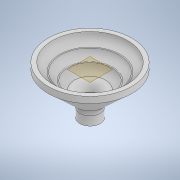
# Autodesk Inventor part: TubeExpander
Saved by Autodesk Inventor 2020 (Build 240168000, 168)
## iProperties
Created: 2020-04-23
Part Number: TubeExpander
Material: Типовые
Document SubType Name: Modeling
Designer: Михаил
Density: 1 g/cm^3
Appearance: По умолчанию
Author: Михаил
Autodesk Inventor part; units mm, degrees
ref_plane "YZ Plane" through (0, 0, 0) normal (1, 0, 0) x (0, 1, 0)
ref_plane "XZ Plane" through (0, 0, 0) normal (0, 1, 0) x (-1, 0, 0)
ref_plane "XY Plane" through (0, 0, 0) normal (0, 0, 1) x (1, 0, 0)
sketch "Эскиз1" plane through (0, 0, 0) normal (0, 1, 0) x (-1, 0, 0)
  circle A0 centre (0, 0) radius 2.45
  dimension "d0" = 4.9
  constraints: 1 centre point, 1 coincident
  measures "d0" diameter of A0
extrude "Выдавливание1" add sketch "Эскиз1" along normal blind 3
ref_plane "РабПлоскость2" through (0, 10, 0) normal (0, 1, 0) x (1, 0, 0)
sketch "Эскиз2" plane through (0, 10, 0) normal (0, 1, 0) x (1, 0, 0)
  circle A0 centre (0, 0) radius 10
  dimension "d4" = 20
  constraints: 1 centre point, 1 coincident
  measures "d4" diameter of A0
extrude "Выдавливание2" add sketch "Эскиз2" along normal blind 1.5
loft "Лофт1" add section 1 edges at (-10, 10, 0) section 2 edges at (2.45, 3, 0)
sketch "Эскиз3" plane through (0, 0, 0) normal (0, -1, 0) x (1, 0, 0)
  circle A0 centre (0, 0) radius 2.45 projected
  circle A1 centre (0, 0) radius 2
  dimension "d11" = 4
  constraints: 1 centre point, 1 coincident
  measures "d11" diameter of A1
sketch "Эскиз4" plane through (0, 0, 0) normal (0, -1, 0) x (1, 0, 0)
  point P0 (0, 0)
extrude "Выдавливание3" cut sketch "Эскиз3" against normal blind 3 contours A1
sketch "Эскиз5" plane through (0, 11.5, 0) normal (0, 1, 0) x (1, 0, 0)
  circle A0 centre (0, 0) radius 9
  dimension "d14" = 18
  constraints: 1 centre point, 1 coincident
  measures "d14" diameter of A0
extrude "Выдавливание4" cut sketch "Эскиз5" against normal blind 2
fillet "Сопряжение1" radius 2 3 edges at (-9, 9.5, 0) (0, 3, -2.45) (0, 3, 2.45)
sketch "Эскиз6" plane through (0, 9.5, 0) normal (0, 1, 0) x (1, 0, 0)
  circle A0 centre (0, 0) radius 7.2679
  constraints: 1 centre point, 1 coincident
extrude "Выдавливание5" cut sketch "Эскиз6" against normal blind 1.8
fillet "Сопряжение2" radius 2 1 edges at (-7.2679, 7.7, 0)
sketch "Эскиз7" plane through (0, 7.7, 0) normal (0, 1, 0) x (1, 0, 0)
  circle A0 centre (0, 0) radius 5.5359
  constraints: 1 centre point, 1 coincident
extrude "Выдавливание6" cut sketch "Эскиз7" against normal blind 1.8
fillet "Сопряжение3" radius 2 1 edges at (-5.5359, 5.9, 0)
sketch "Эскиз11" plane through (0, 5.9, 0) normal (0, 1, 0) x (1, 0, 0)
  circle A0 centre (0, 0) radius 2
  constraints: 1 centre point, 1 coincident
extrude "Выдавливание10" cut sketch "Эскиз11" against normal blind 3.1
fillet "Сопряжение6" radius 2 1 edges at (-2, 5.9, 0)
